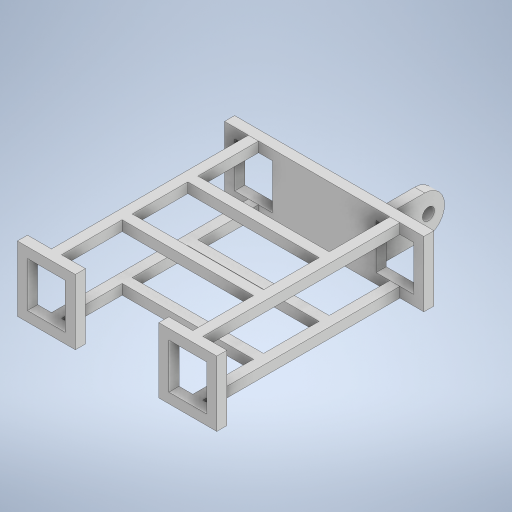
# Autodesk Inventor part: MHead
Saved by Autodesk Inventor 2024 (Build 280153000, 153)
## iProperties
Created: 2023-06-14
Part Number: MHead
Material: Generic
Document SubType Name: Modeling
Designer: vilas
Density: 1 g/cm^3
Appearance: Default
Author: vilas
Autodesk Inventor part; units mm, degrees
ref_plane "YZ Plane" through (0, 0, 0) normal (1, 0, 0) x (0, 1, 0)
sketch "Sketch1" plane through (0, 0, 0) normal (0, 0, 1) x (1, 0, 0)
  line L0 (-32.5, 11.15) -> (32.5, 11.15) construction
  line L1 (32.5, 11.15) -> (32.5, -11.15) construction
  line L2 (32.5, -11.15) -> (-32.5, -11.15) construction
  line L3 (-32.5, -11.15) -> (-32.5, 11.15) construction
  line L4 (-32.5, 11.15) -> (32.5, -11.15) construction
  line L5 (32.5, 11.15) -> (-32.5, -11.15) construction
  line L6 (-32.5, 11.15) -> (-37.5, 11.15)
  line L7 (-37.5, 11.15) -> (-37.5, 16.15)
  line L8 (-37.5, 16.15) -> (-32.5, 16.15)
  line L9 (-32.5, 16.15) -> (-32.5, 11.15)
  line L10 (32.5, 11.15) -> (37.5, 11.15)
  line L11 (37.5, 11.15) -> (37.5, 16.15)
  line L12 (37.5, 16.15) -> (32.5, 16.15)
  line L13 (32.5, 16.15) -> (32.5, 11.15)
  line L14 (32.5, -11.15) -> (37.5, -11.15)
  line L15 (37.5, -11.15) -> (37.5, -16.15)
  line L16 (37.5, -16.15) -> (32.5, -16.15)
  line L17 (32.5, -16.15) -> (32.5, -11.15)
  line L18 (-32.5, -11.15) -> (-37.5, -11.15)
  line L19 (-37.5, -11.15) -> (-37.5, -16.15)
  line L20 (-37.5, -16.15) -> (-32.5, -16.15)
  line L21 (-32.5, -16.15) -> (-32.5, -11.15)
  point P0 (0, 0)
  dimension "d0" = 65
  dimension "d1" = 22.3
  dimension "d2" = 5
  dimension "d3" = 5
  dimension "d4" = 5
  dimension "d5" = 5
  dimension "d6" = 5
  dimension "d7" = 5
  dimension "d8" = 5
  dimension "d9" = 5
  constraints: 44 end point, 10 parallel, 5 horizontal, 5 perpendicular, 2 midpoint
  measures "d0" distance of L1.end L2.end
  measures "d1" distance of L0.end L1.end
  measures "d2" distance of L7.end L8.end
  measures "d3" distance of L6.end L7.end
  measures "d4" distance of L12.end L11.end
  measures "d5" distance of L11.end L10.end
  measures "d6" distance of L15.end L16.end
  measures "d7" distance of L14.end L15.end
  measures "d8" distance of L20.end L19.end
  measures "d9" distance of L19.end L18.end
extrude "Extrusion1" add sketch "Sketch1" along normal mid plane 97.524
ref_plane "Work Plane1" through (0, 0, 48.762) normal (0, 0, 1) x (1, 0, 0)
sketch "Sketch2" plane through (0, 0, 48.762) normal (0, 0, 1) x (1, 0, 0)
  line L0 (0, 0) -> (-35, 0) construction
  line L1 (0, 0) -> (35, 0) construction
  line L2 (-49.35, 16.15) -> (-20.65, 16.15)
  line L3 (-20.65, 16.15) -> (-20.65, -16.15)
  line L4 (-20.65, -16.15) -> (-49.35, -16.15)
  line L5 (-49.35, -16.15) -> (-49.35, 16.15)
  line L6 (-49.35, 16.15) -> (-20.65, -16.15) construction
  line L7 (-20.65, 16.15) -> (-49.35, -16.15) construction
  line L8 (20.65, 16.15) -> (49.35, 16.15)
  line L9 (49.35, 16.15) -> (49.35, -16.15)
  line L10 (49.35, -16.15) -> (20.65, -16.15)
  line L11 (20.65, -16.15) -> (20.65, 16.15)
  line L12 (20.65, 16.15) -> (49.35, -16.15) construction
  line L13 (49.35, 16.15) -> (20.65, -16.15) construction
  line L14 (-25.65, 11.15) -> (-44.35, 11.15)
  line L15 (-44.35, 11.15) -> (-44.35, -11.15)
  line L16 (-44.35, -11.15) -> (-25.65, -11.15)
  line L17 (-25.65, -11.15) -> (-25.65, 11.15)
  line L18 (44.35, 11.15) -> (25.65, 11.15)
  line L19 (25.65, 11.15) -> (25.65, -11.15)
  line L20 (25.65, -11.15) -> (44.35, -11.15)
  line L21 (44.35, -11.15) -> (44.35, 11.15)
  dimension "d13" = 35
  dimension "d14" = 35
  dimension "d15" = 28.7
  dimension "d16" = 32.3
  dimension "d17" = 28.7
  dimension "d18" = 32.3
  dimension "d19" = 5
  dimension "d20" = 5
  constraints: 44 end point, 8 parallel, 4 horizontal, 4 midpoint, 4 perpendicular, 6 other
  measures "d13" distance of L0.start L0.end
  measures "d14" distance of L0.start L1.end
  measures "d15" distance of L3.end L4.end
  measures "d16" distance of L2.end L3.end
  measures "d17" distance of L9.end L10.end
  measures "d18" distance of L8.end L9.end
  measures "d19" distance between parallel lines of L2 L14
  measures "d20" distance between parallel lines of L8 L18
extrude "Extrusion2" add sketch "Sketch2" along normal blind 5
ref_plane "Work Plane2" through (0, 0, -48.771) normal (0, 0, 1) x (1, 0, 0)
sketch "Sketch3" plane through (0, 0, -48.771) normal (0, 0, 1) x (1, 0, 0)
  line L0 (49.35, 16.15) -> (-49.35, 16.15)
  line L1 (-49.35, 16.15) -> (-49.35, -16.15)
  line L2 (-49.35, -16.15) -> (49.35, -16.15)
  line L3 (49.35, -16.15) -> (49.35, 16.15)
  line L4 (49.35, 16.15) -> (-49.35, -16.15) construction
  line L5 (-49.35, 16.15) -> (49.35, -16.15) construction
  line L6 (0, 0) -> (35, 0) construction
  line L7 (0, 0) -> (-35, 0) construction
  line L8 (32.5, -11.15) -> (25.65, -11.15) projected
  line L9 (44.35, 11.15) -> (25.65, 11.15)
  line L10 (25.65, 11.15) -> (25.65, -11.15)
  line L11 (25.65, -11.15) -> (44.35, -11.15)
  line L12 (44.35, -11.15) -> (44.35, 11.15)
  line L13 (44.35, 11.15) -> (25.65, -11.15) construction
  line L14 (25.65, 11.15) -> (44.35, -11.15) construction
  line L15 (-44.35, -11.15) -> (-44.35, 11.15) projected
  line L16 (-25.65, -11.15) -> (-44.35, -11.15)
  line L17 (-44.35, -11.15) -> (-44.35, 11.15)
  line L18 (-44.35, 11.15) -> (-25.65, 11.15)
  line L19 (-25.65, 11.15) -> (-25.65, -11.15)
  line L20 (-25.65, -11.15) -> (-44.35, 11.15) construction
  line L21 (-44.35, -11.15) -> (-25.65, 11.15) construction
  point P0 (30, -11.15)
  dimension "d24" = 98.7
  dimension "d25" = 32.3
  dimension "d26" = 35
  dimension "d27" = 35
  constraints: 40 end point, 6 midpoint, 6 parallel, 4 horizontal, 3 perpendicular, 1 point on line
  measures "d24" distance of L2.end L1.end
  measures "d25" distance of L1.end L0.end
  measures "d26" distance of L6.start L6.end
  measures "d27" distance of L6.start L7.end
extrude "Extrusion3" add sketch "Sketch3" against normal blind 5
sketch "Sketch4" plane through (0, 0, 0) normal (1, 0, 0) x (0, 1, 0)
  line L0 (11.15, -48.762) -> (11.15, 48.762) projected
  line L1 (11.15, 18.754) -> (16.15, 18.754)
  line L2 (16.15, 18.754) -> (16.15, 13.754)
  line L3 (16.15, 13.754) -> (11.15, 13.754)
  line L4 (11.15, 13.754) -> (11.15, 18.754)
  line L5 (-16.15, 48.762) -> (16.15, 48.762) projected
  line L6 (11.15, -13.754) -> (16.15, -13.754)
  line L7 (16.15, -13.754) -> (16.15, -18.754)
  line L8 (16.15, -18.754) -> (11.15, -18.754)
  line L9 (11.15, -18.754) -> (11.15, -13.754)
  line L10 (16.15, -48.762) -> (11.15, -48.762) projected
  line L11 (-11.15, 48.762) -> (-11.15, -48.762) projected
  line L12 (-11.15, 18.754) -> (-16.15, 18.754)
  line L13 (-16.15, 18.754) -> (-16.15, 13.754)
  line L14 (-16.15, 13.754) -> (-11.15, 13.754)
  line L15 (-11.15, 13.754) -> (-11.15, 18.754)
  line L16 (-11.15, -18.754) -> (-16.15, -18.754)
  line L17 (-16.15, -18.754) -> (-16.15, -13.754)
  line L18 (-16.15, -13.754) -> (-11.15, -13.754)
  line L19 (-11.15, -13.754) -> (-11.15, -18.754)
  line L20 (-11.15, -48.762) -> (-16.15, -48.762) projected
  point P0 (0, 0)
  dimension "d30" = 5
  dimension "d31" = 5
  dimension "d32" = 30.008
  dimension "d33" = 5
  dimension "d34" = 5
  dimension "d35" = 30.008
  dimension "d36" = 5
  dimension "d37" = 5
  dimension "d38" = 5
  dimension "d39" = 5
  dimension "d40" = 30.008
  dimension "d41" = 30.008
  constraints: 32 end point, 8 parallel, 4 horizontal, 4 perpendicular, 4 point on line
  measures "d30" distance of L2.end L3.end
  measures "d31" distance of L1.end L2.end
  measures "d32" distance between parallel lines of L1 L5
  measures "d33" distance of L7.end L8.end
  measures "d34" distance of L6.end L7.end
  measures "d35" distance between parallel lines of L8 L10
  measures "d36" distance of L14.end L13.end
  measures "d37" distance of L13.end L12.end
  measures "d38" distance of L17.end L18.end
  measures "d39" distance of L16.end L17.end
  measures "d40" distance between parallel lines of L16 L20
  measures "d41" distance between parallel lines of L12 L5
extrude "Extrusion4" add sketch "Sketch4" along normal mid plane 65
sketch "Sketch5" plane through (0, 0, -53.771) normal (0, 0, -1) x (-1, 0, 0)
  line L0 (-24.603, 9.85) -> (-19.603, 9.85)
  line L1 (-19.603, 9.85) -> (-19.603, -9.85)
  line L2 (-19.603, -9.85) -> (-24.603, -9.85)
  line L3 (-24.603, -9.85) -> (-24.603, 9.85)
  line L4 (-24.603, 9.85) -> (-19.603, -9.85) construction
  line L5 (-19.603, 9.85) -> (-24.603, -9.85) construction
  point P0 (0, 0)
  point P1 (-22.103, 0)
  dimension "d44" = 5
  dimension "d45" = 19.7
  dimension "d46" = 24.603
  constraints: 12 end point, 2 midpoint, 2 parallel, 1 horizontal, 1 perpendicular
  measures "d44" distance of L1.end L2.end
  measures "d45" distance of L0.end L1.end
  measures "d46" distance from line of L3 point (0, 0)
extrude "Extrusion5" add sketch "Sketch5" along normal blind 30
fillet "Fillet1" radius 9.85 2 edges at (22.103, 9.85, -83.771) (22.103, -9.85, -83.771)
sketch "Sketch6" plane through (19.603, -9.85, -53.771) normal (-1, 0, 0) x (0, 0, 1)
  line L0 (0, -1.3) -> (0, 21) construction
  line L1 (0, 9.85) -> (-22, 9.85) construction
  circle A0 centre (-22, 9.85) radius 3
  point P0 (53.771, 9.85)
  dimension "d50" = 22
  dimension "d51" = 6
  constraints: 2 end point, 1 centre point, 1 coincident, 1 horizontal, 1 midpoint
  measures "d50" distance of L1.start L1.end
  measures "d51" diameter of A0
extrude "Extrusion6" cut sketch "Sketch6" against normal through all
body "Solid1"
